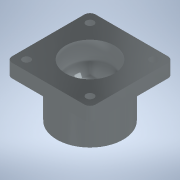
# Autodesk Inventor part: Soporte
Saved by Autodesk Inventor 2022.1 (Build 261234000, 234)
## iProperties
Part Number: Soporte
Material: Genérico
Document SubType Name: Modelado
Designer: seb_0
Appearance: Zinc
Author: seb_0
Autodesk Inventor part; units mm, degrees
ref_plane "Plano YZ" through (0, 0, 0) normal (1, 0, 0) x (0, 1, 0)
ref_plane "Plano XZ" through (0, 0, 0) normal (0, 1, 0) x (-1, 0, 0)
ref_plane "Plano XY" through (0, 0, 0) normal (0, 0, 1) x (1, 0, 0)
sketch "Boceto1" plane through (0, 0, 0) normal (0, 1, 0) x (-1, 0, 0)
  circle A0 centre (0, 0) radius 30.25
  dimension "d0" = 60.5
  constraints: 1 centre point, 1 coincident
  measures "d0" diameter of A0
extrude "Extrusión1" add sketch "Boceto1" along normal blind 48.2
sketch "Boceto2" plane through (0, 48.2, 0) normal (0, 1, 0) x (1, 0, 0)
  line L0 (-38.1, -38.1) -> (38.1, -38.1)
  line L1 (38.1, -38.1) -> (38.1, 38.1)
  line L2 (38.1, 38.1) -> (-38.1, 38.1)
  line L3 (-38.1, 38.1) -> (-38.1, -38.1)
  line L4 (38.1, -38.1) -> (-38.1, 38.1)
  line L5 (38.1, 38.1) -> (-38.1, -38.1)
  point P0 (0, 0)
  point P1 (0, 0)
  dimension "d3" = 76.2
  constraints: 12 end point, 3 perpendicular, 2 parallel, 1 coincident, 1 horizontal, 1 midpoint
  measures "d3" distance of L2.end L0.start
extrude "Extrusión2" add sketch "Boceto2" against normal blind 12.4
sketch "Boceto3" plane through (0, 48.2, 0) normal (0, 1, 0) x (1, 0, 0)
  line L0 (-38.1, 38.1) -> (-38.1, -38.1) projected
  line L1 (-38.1, -38.1) -> (38.1, -38.1) projected
  line L2 (38.1, -38.1) -> (38.1, 38.1) projected
  line L3 (38.1, 38.1) -> (-38.1, 38.1) projected
  line L4 (-28.95, -28.95) -> (-28.95, 28.95)
  line L5 (-28.95, 28.95) -> (28.95, 28.95)
  line L6 (28.95, 28.95) -> (28.95, -28.95)
  line L7 (28.95, -28.95) -> (-28.95, -28.95)
  circle A0 centre (-28.95, -28.95) radius 3.55
  circle A1 centre (-28.95, 28.95) radius 3.55
  circle A2 centre (28.95, 28.95) radius 3.55
  circle A3 centre (28.95, -28.95) radius 3.55
  dimension "d7" = 57.9
  dimension "d8" = 7.1
  constraints: 8 end point, 4 centre point, 4 coincident, 3 equal radius, 3 other
  measures "d7" distance of L4.start L4.end
  measures "d8" diameter of A0
extrude "Extrusión3" cut sketch "Boceto3" against normal through all contours L7 A0 L4 | L4 A0 L7 | A1 L5 L4 | L4 L5 A1 | A3 L6 L7 | L7 L6 A3 | A2 L6 L5 | L5 L6 A2
fillet "Empalme1" radius 5 4 edges at (38.1, 42, 38.1) (38.1, 42, -38.1) (-38.1, 42, 38.1) (-38.1, 42, -38.1)
ref_plane "Plano de trabajo1" through (0, 35.8, 0) normal (0, -1, 0) x (1, 0, 0)
sketch "Boceto4" plane through (0, 35.8, 0) normal (0, -1, 0) x (1, 0, 0)
  circle A0 centre (0, 0) radius 25.4
  line L0 (0, 25.4) -> (0, -25.4)
  dimension "d13" = 50.8
  constraints: 2 end point, 2 point on circle, 1 centre point, 1 coincident, 1 vertical
  measures "d13" diameter of A0
revolve "Revolución1" cut sketch "Boceto4" angle 360 about axis through (0, 35.8, 25.4) along (0, 0, -1) picked at (5.2789, 6.6195) contours A0 L0
